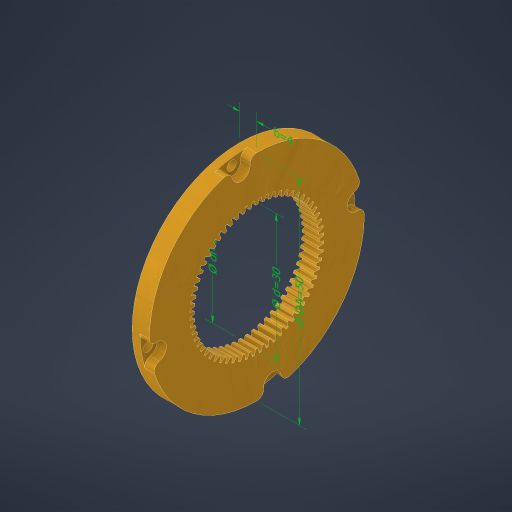
# Autodesk Inventor part: 60z
Saved by Autodesk Inventor 2024.1 (Build 281209000, 209)
## iProperties
Category: PARTsolutions
Company: MAEDLER
Created: 2023-10-17
Part Number: 60z
Material: Generic
Catalog Web Link: www.cadenas.de
Description: MAE-IZK-M0.5-MS58-Straight-Toothed Internal Gears Made from Brass MS58, Module 0,5
Vendor: MAEDLER
Document SubType Name: Modeling
Designer: psAdmin
Manufacturer: MAEDLER
Mass: 42 g
Surface Area: 39.2862 cm^2
Volume: 5.00767 cm^3
Density: 1 g/cm^3
Appearance: Schweißnaht - Messing
PSOL_IDENT_0: {$CADENAS_DATA/23d-libs/maedler/antriebselemente/innenzahnkraenze/innenzahnkr_m0_5_ms58.prj},167 {VT
PSOL_IDENT_1: YP=3D},{NB=26146000},{LINA=26146000},{NN=MAE-IZK-M0.5-MS58},{DATE=12.10.2023 13:22:54},{GEOMDATE=09.
PSOL_IDENT_2: 07.2023 12:07:43},{VERSION=},{LINEID=50},{WBVAR=},{WBNUMERIC=}  {NB=26146000},{LINA=26146000},{KT=DU
PSOL_IDENT_3: MMY},{ARTNR=26146000},{WEBSHOP=Produktdetails / Katalogseite / Montageanleitung},{MAT=Messing MS58 (
PSOL_IDENT_4: 2.0401)},{M=0.5},{Z=60},{B=4},{D=30.0},{DI=29.0},{DA=50},{GEW=42},{ZTN=84839089},{DIST=1.800}
NB: 26146000
NN: MAE-IZK-M0.5-MS58
NT: Straight-Toothed Internal Gears Made from Brass MS58, Module 0,5
NBSYN: $ARTNR.
LINA: 26146000
CATALOG: Mädler
ARTNR: 26146000
WEBSHOP: Product details / Catalogue page / Assembly instructions
MAT: Brass Ms58 (2.0401)
M: 0.5
Z: 60
B: 4
D: 30
DI: 29
DA: 50
GEW: 42
ZTN: 84839089
SUPPLIER: MAEDLER
ARTICLENO: 26146000
BOMINFO: 26146000
CREATOR: CADENAS GmbH
Title: 26146000
Author: Cadenas PARTsolutions
Comments: Straight-Toothed Internal Gears Made from Brass MS58, Module 0,5
Autodesk Inventor part; units mm, degrees
ref_plane "YZ Plane" through (0, 0, 0) normal (1, 0, 0) x (0, 1, 0)
ref_plane "XZ Plane" through (0, 0, 0) normal (0, 1, 0) x (-1, 0, 0)
ref_plane "XY Plane" through (0, 0, 0) normal (0, 0, 1) x (1, 0, 0)
sketch "Skizze_1" plane through (0, 0, 0) normal (1, 0, 0) x (0, 1, 0)
  circle A0 centre (0, 0) radius 25
  line L0 (0.5705, 15.6146) -> (0.25, 14.4978)
  arc A1 (0.25, 14.4978) -> (-0.25, 14.4978) centre (0, 0) ccw
  line L1 (-0.25, 14.4978) -> (-0.5705, 15.6146)
  arc A2 (-0.5705, 15.6146) -> (-1.0648, 15.5887) centre (0, 0) ccw
  line L2 (-1.0648, 15.5887) -> (-1.2668, 14.4446)
  arc A3 (-1.2668, 14.4446) -> (-1.7641, 14.3923) centre (0, 0) ccw
  line L3 (-1.7641, 14.3923) -> (-2.1996, 15.4694)
  arc A4 (-2.1996, 15.4694) -> (-2.6884, 15.392) centre (0, 0) ccw
  line L4 (-2.6884, 15.392) -> (-2.7697, 14.233)
  arc A5 (-2.7697, 14.233) -> (-3.2588, 14.1291) centre (0, 0) ccw
  line L5 (-3.2588, 14.1291) -> (-3.8045, 15.1547)
  arc A6 (-3.8045, 15.1547) -> (-4.2826, 15.0267) centre (0, 0) ccw
  line L6 (-4.2826, 15.0267) -> (-4.2423, 13.8655)
  arc A7 (-4.2423, 13.8655) -> (-4.7178, 13.711) centre (0, 0) ccw
  line L7 (-4.7178, 13.711) -> (-5.3678, 14.674)
  arc A8 (-5.3678, 14.674) -> (-5.8298, 14.4967) centre (0, 0) ccw
  line L8 (-5.8298, 14.4967) -> (-5.6684, 13.3461)
  arc A9 (-5.6684, 13.3461) -> (-6.1252, 13.1428) centre (0, 0) ccw
  line L9 (-6.1252, 13.1428) -> (-6.8722, 14.0326)
  arc A10 (-6.8722, 14.0326) -> (-7.3132, 13.8079) centre (0, 0) ccw
  line L10 (-7.3132, 13.8079) -> (-7.0324, 12.6805)
  arc A11 (-7.0324, 12.6805) -> (-7.4654, 12.4305) centre (0, 0) ccw
  line L11 (-7.4654, 12.4305) -> (-8.3014, 13.2374)
  arc A12 (-8.3014, 13.2374) -> (-8.7165, 12.9678) centre (0, 0) ccw
  line L12 (-8.7165, 12.9678) -> (-8.3194, 11.8759)
  arc A13 (-8.3194, 11.8759) -> (-8.7239, 11.5821) centre (0, 0) ccw
  line L13 (-8.7239, 11.5821) -> (-9.6396, 12.2971)
  arc A14 (-9.6396, 12.2971) -> (-10.0242, 11.9857) centre (0, 0) ccw
  line L14 (-10.0242, 11.9857) -> (-9.5152, 10.9413)
  arc A15 (-9.5152, 10.9413) -> (-9.8867, 10.6067) centre (0, 0) ccw
  line L15 (-9.8867, 10.6067) -> (-10.8722, 11.2221)
  arc A16 (-10.8722, 11.2221) -> (-11.2221, 10.8722) centre (0, 0) ccw
  line L16 (-11.2221, 10.8722) -> (-10.6067, 9.8867)
  arc A17 (-10.6067, 9.8867) -> (-10.9413, 9.5152) centre (0, 0) ccw
  line L17 (-10.9413, 9.5152) -> (-11.9857, 10.0242)
  arc A18 (-11.9857, 10.0242) -> (-12.2971, 9.6396) centre (0, 0) ccw
  line L18 (-12.2971, 9.6396) -> (-11.5821, 8.7239)
  arc A19 (-11.5821, 8.7239) -> (-11.8759, 8.3194) centre (0, 0) ccw
  line L19 (-11.8759, 8.3194) -> (-12.9678, 8.7165)
  arc A20 (-12.9678, 8.7165) -> (-13.2374, 8.3014) centre (0, 0) ccw
  line L20 (-13.2374, 8.3014) -> (-12.4305, 7.4654)
  arc A21 (-12.4305, 7.4654) -> (-12.6805, 7.0324) centre (0, 0) ccw
  line L21 (-12.6805, 7.0324) -> (-13.8079, 7.3132)
  arc A22 (-13.8079, 7.3132) -> (-14.0326, 6.8722) centre (0, 0) ccw
  line L22 (-14.0326, 6.8722) -> (-13.1428, 6.1252)
  arc A23 (-13.1428, 6.1252) -> (-13.3461, 5.6684) centre (0, 0) ccw
  line L23 (-13.3461, 5.6684) -> (-14.4967, 5.8298)
  arc A24 (-14.4967, 5.8298) -> (-14.674, 5.3678) centre (0, 0) ccw
  line L24 (-14.674, 5.3678) -> (-13.711, 4.7178)
  arc A25 (-13.711, 4.7178) -> (-13.8655, 4.2423) centre (0, 0) ccw
  line L25 (-13.8655, 4.2423) -> (-15.0267, 4.2826)
  arc A26 (-15.0267, 4.2826) -> (-15.1547, 3.8045) centre (0, 0) ccw
  line L26 (-15.1547, 3.8045) -> (-14.1291, 3.2588)
  arc A27 (-14.1291, 3.2588) -> (-14.233, 2.7697) centre (0, 0) ccw
  line L27 (-14.233, 2.7697) -> (-15.392, 2.6884)
  arc A28 (-15.392, 2.6884) -> (-15.4694, 2.1996) centre (0, 0) ccw
  line L28 (-15.4694, 2.1996) -> (-14.3923, 1.7641)
  arc A29 (-14.3923, 1.7641) -> (-14.4446, 1.2668) centre (0, 0) ccw
  line L29 (-14.4446, 1.2668) -> (-15.5887, 1.0648)
  arc A30 (-15.5887, 1.0648) -> (-15.6146, 0.5705) centre (0, 0) ccw
  line L30 (-15.6146, 0.5705) -> (-14.4978, 0.25)
  arc A31 (-14.4978, 0.25) -> (-14.4978, -0.25) centre (0, 0) ccw
  line L31 (-14.4978, -0.25) -> (-15.6146, -0.5705)
  arc A32 (-15.6146, -0.5705) -> (-15.5887, -1.0648) centre (0, 0) ccw
  line L32 (-15.5887, -1.0648) -> (-14.4446, -1.2668)
  arc A33 (-14.4446, -1.2668) -> (-14.3923, -1.7641) centre (0, 0) ccw
  line L33 (-14.3923, -1.7641) -> (-15.4694, -2.1996)
  arc A34 (-15.4694, -2.1996) -> (-15.392, -2.6884) centre (0, 0) ccw
  line L34 (-15.392, -2.6884) -> (-14.233, -2.7697)
  arc A35 (-14.233, -2.7697) -> (-14.1291, -3.2588) centre (0, 0) ccw
  line L35 (-14.1291, -3.2588) -> (-15.1547, -3.8045)
  arc A36 (-15.1547, -3.8045) -> (-15.0267, -4.2826) centre (0, 0) ccw
  line L36 (-15.0267, -4.2826) -> (-13.8655, -4.2423)
  arc A37 (-13.8655, -4.2423) -> (-13.711, -4.7178) centre (0, 0) ccw
  line L37 (-13.711, -4.7178) -> (-14.674, -5.3678)
  arc A38 (-14.674, -5.3678) -> (-14.4967, -5.8298) centre (0, 0) ccw
  line L38 (-14.4967, -5.8298) -> (-13.3461, -5.6684)
  arc A39 (-13.3461, -5.6684) -> (-13.1428, -6.1252) centre (0, 0) ccw
  line L39 (-13.1428, -6.1252) -> (-14.0326, -6.8722)
  arc A40 (-14.0326, -6.8722) -> (-13.8079, -7.3132) centre (0, 0) ccw
  line L40 (-13.8079, -7.3132) -> (-12.6805, -7.0324)
  arc A41 (-12.6805, -7.0324) -> (-12.4305, -7.4654) centre (0, 0) ccw
  line L41 (-12.4305, -7.4654) -> (-13.2374, -8.3014)
  arc A42 (-13.2374, -8.3014) -> (-12.9678, -8.7165) centre (0, 0) ccw
  line L42 (-12.9678, -8.7165) -> (-11.8759, -8.3194)
  arc A43 (-11.8759, -8.3194) -> (-11.5821, -8.7239) centre (0, 0) ccw
  line L43 (-11.5821, -8.7239) -> (-12.2971, -9.6396)
  arc A44 (-12.2971, -9.6396) -> (-11.9857, -10.0242) centre (0, 0) ccw
  line L44 (-11.9857, -10.0242) -> (-10.9413, -9.5152)
  arc A45 (-10.9413, -9.5152) -> (-10.6067, -9.8867) centre (0, 0) ccw
  line L45 (-10.6067, -9.8867) -> (-11.2221, -10.8722)
  arc A46 (-11.2221, -10.8722) -> (-10.8722, -11.2221) centre (0, 0) ccw
  line L46 (-10.8722, -11.2221) -> (-9.8867, -10.6067)
  arc A47 (-9.8867, -10.6067) -> (-9.5152, -10.9413) centre (0, 0) ccw
  line L47 (-9.5152, -10.9413) -> (-10.0242, -11.9857)
  arc A48 (-10.0242, -11.9857) -> (-9.6396, -12.2971) centre (0, 0) ccw
  line L48 (-9.6396, -12.2971) -> (-8.7239, -11.5821)
  arc A49 (-8.7239, -11.5821) -> (-8.3194, -11.8759) centre (0, 0) ccw
  line L49 (-8.3194, -11.8759) -> (-8.7165, -12.9678)
  arc A50 (-8.7165, -12.9678) -> (-8.3014, -13.2374) centre (0, 0) ccw
  line L50 (-8.3014, -13.2374) -> (-7.4654, -12.4305)
  arc A51 (-7.4654, -12.4305) -> (-7.0324, -12.6805) centre (0, 0) ccw
  line L51 (-7.0324, -12.6805) -> (-7.3132, -13.8079)
  arc A52 (-7.3132, -13.8079) -> (-6.8722, -14.0326) centre (0, 0) ccw
  line L52 (-6.8722, -14.0326) -> (-6.1252, -13.1428)
  arc A53 (-6.1252, -13.1428) -> (-5.6684, -13.3461) centre (0, 0) ccw
  line L53 (-5.6684, -13.3461) -> (-5.8298, -14.4967)
  arc A54 (-5.8298, -14.4967) -> (-5.3678, -14.674) centre (0, 0) ccw
  line L54 (-5.3678, -14.674) -> (-4.7178, -13.711)
  arc A55 (-4.7178, -13.711) -> (-4.2423, -13.8655) centre (0, 0) ccw
  line L55 (-4.2423, -13.8655) -> (-4.2826, -15.0267)
  arc A56 (-4.2826, -15.0267) -> (-3.8045, -15.1547) centre (0, 0) ccw
  line L56 (-3.8045, -15.1547) -> (-3.2588, -14.1291)
  arc A57 (-3.2588, -14.1291) -> (-2.7697, -14.233) centre (0, 0) ccw
  line L57 (-2.7697, -14.233) -> (-2.6884, -15.392)
  arc A58 (-2.6884, -15.392) -> (-2.1996, -15.4694) centre (0, 0) ccw
  line L58 (-2.1996, -15.4694) -> (-1.7641, -14.3923)
  arc A59 (-1.7641, -14.3923) -> (-1.2668, -14.4446) centre (0, 0) ccw
  line L59 (-1.2668, -14.4446) -> (-1.0648, -15.5887)
  arc A60 (-1.0648, -15.5887) -> (-0.5705, -15.6146) centre (0, 0) ccw
  line L60 (-0.5705, -15.6146) -> (-0.25, -14.4978)
  arc A61 (-0.25, -14.4978) -> (0.25, -14.4978) centre (0, 0) ccw
  line L61 (0.25, -14.4978) -> (0.5705, -15.6146)
  arc A62 (0.5705, -15.6146) -> (1.0648, -15.5887) centre (0, 0) ccw
  line L62 (1.0648, -15.5887) -> (1.2668, -14.4446)
  arc A63 (1.2668, -14.4446) -> (1.7641, -14.3923) centre (0, 0) ccw
  line L63 (1.7641, -14.3923) -> (2.1996, -15.4694)
  arc A64 (2.1996, -15.4694) -> (2.6884, -15.392) centre (0, 0) ccw
  line L64 (2.6884, -15.392) -> (2.7697, -14.233)
  arc A65 (2.7697, -14.233) -> (3.2588, -14.1291) centre (0, 0) ccw
  line L65 (3.2588, -14.1291) -> (3.8045, -15.1547)
  arc A66 (3.8045, -15.1547) -> (4.2826, -15.0267) centre (0, 0) ccw
  line L66 (4.2826, -15.0267) -> (4.2423, -13.8655)
  arc A67 (4.2423, -13.8655) -> (4.7178, -13.711) centre (0, 0) ccw
  line L67 (4.7178, -13.711) -> (5.3678, -14.674)
  arc A68 (5.3678, -14.674) -> (5.8298, -14.4967) centre (0, 0) ccw
  line L68 (5.8298, -14.4967) -> (5.6684, -13.3461)
  arc A69 (5.6684, -13.3461) -> (6.1252, -13.1428) centre (0, 0) ccw
  line L69 (6.1252, -13.1428) -> (6.8722, -14.0326)
  arc A70 (6.8722, -14.0326) -> (7.3132, -13.8079) centre (0, 0) ccw
  line L70 (7.3132, -13.8079) -> (7.0324, -12.6805)
  arc A71 (7.0324, -12.6805) -> (7.4654, -12.4305) centre (0, 0) ccw
  line L71 (7.4654, -12.4305) -> (8.3014, -13.2374)
  arc A72 (8.3014, -13.2374) -> (8.7165, -12.9678) centre (0, 0) ccw
  line L72 (8.7165, -12.9678) -> (8.3194, -11.8759)
  arc A73 (8.3194, -11.8759) -> (8.7239, -11.5821) centre (0, 0) ccw
  line L73 (8.7239, -11.5821) -> (9.6396, -12.2971)
  arc A74 (9.6396, -12.2971) -> (10.0242, -11.9857) centre (0, 0) ccw
  line L74 (10.0242, -11.9857) -> (9.5152, -10.9413)
  arc A75 (9.5152, -10.9413) -> (9.8867, -10.6067) centre (0, 0) ccw
  line L75 (9.8867, -10.6067) -> (10.8722, -11.2221)
  arc A76 (10.8722, -11.2221) -> (11.2221, -10.8722) centre (0, 0) ccw
  line L76 (11.2221, -10.8722) -> (10.6067, -9.8867)
  arc A77 (10.6067, -9.8867) -> (10.9413, -9.5152) centre (0, 0) ccw
  line L77 (10.9413, -9.5152) -> (11.9857, -10.0242)
  arc A78 (11.9857, -10.0242) -> (12.2971, -9.6396) centre (0, 0) ccw
  line L78 (12.2971, -9.6396) -> (11.5821, -8.7239)
  arc A79 (11.5821, -8.7239) -> (11.8759, -8.3194) centre (0, 0) ccw
  line L79 (11.8759, -8.3194) -> (12.9678, -8.7165)
  arc A80 (12.9678, -8.7165) -> (13.2374, -8.3014) centre (0, 0) ccw
  line L80 (13.2374, -8.3014) -> (12.4305, -7.4654)
  arc A81 (12.4305, -7.4654) -> (12.6805, -7.0324) centre (0, 0) ccw
  line L81 (12.6805, -7.0324) -> (13.8079, -7.3132)
  arc A82 (13.8079, -7.3132) -> (14.0326, -6.8722) centre (0, 0) ccw
  line L82 (14.0326, -6.8722) -> (13.1428, -6.1252)
  arc A83 (13.1428, -6.1252) -> (13.3461, -5.6684) centre (0, 0) ccw
  line L83 (13.3461, -5.6684) -> (14.4967, -5.8298)
  arc A84 (14.4967, -5.8298) -> (14.674, -5.3678) centre (0, 0) ccw
  line L84 (14.674, -5.3678) -> (13.711, -4.7178)
  arc A85 (13.711, -4.7178) -> (13.8655, -4.2423) centre (0, 0) ccw
  line L85 (13.8655, -4.2423) -> (15.0267, -4.2826)
  arc A86 (15.0267, -4.2826) -> (15.1547, -3.8045) centre (0, 0) ccw
  line L86 (15.1547, -3.8045) -> (14.1291, -3.2588)
  arc A87 (14.1291, -3.2588) -> (14.233, -2.7697) centre (0, 0) ccw
  line L87 (14.233, -2.7697) -> (15.392, -2.6884)
  arc A88 (15.392, -2.6884) -> (15.4694, -2.1996) centre (0, 0) ccw
  line L88 (15.4694, -2.1996) -> (14.3923, -1.7641)
  arc A89 (14.3923, -1.7641) -> (14.4446, -1.2668) centre (0, 0) ccw
  line L89 (14.4446, -1.2668) -> (15.5887, -1.0648)
  arc A90 (15.5887, -1.0648) -> (15.6146, -0.5705) centre (0, 0) ccw
  line L90 (15.6146, -0.5705) -> (14.4978, -0.25)
  arc A91 (14.4978, -0.25) -> (14.4978, 0.25) centre (0, 0) ccw
  line L91 (14.4978, 0.25) -> (15.6146, 0.5705)
  arc A92 (15.6146, 0.5705) -> (15.5887, 1.0648) centre (0, 0) ccw
  line L92 (15.5887, 1.0648) -> (14.4446, 1.2668)
  arc A93 (14.4446, 1.2668) -> (14.3923, 1.7641) centre (0, 0) ccw
  line L93 (14.3923, 1.7641) -> (15.4694, 2.1996)
  arc A94 (15.4694, 2.1996) -> (15.392, 2.6884) centre (0, 0) ccw
  line L94 (15.392, 2.6884) -> (14.233, 2.7697)
  arc A95 (14.233, 2.7697) -> (14.1291, 3.2588) centre (0, 0) ccw
  line L95 (14.1291, 3.2588) -> (15.1547, 3.8045)
  arc A96 (15.1547, 3.8045) -> (15.0267, 4.2826) centre (0, 0) ccw
  line L96 (15.0267, 4.2826) -> (13.8655, 4.2423)
  arc A97 (13.8655, 4.2423) -> (13.711, 4.7178) centre (0, 0) ccw
  line L97 (13.711, 4.7178) -> (14.674, 5.3678)
  arc A98 (14.674, 5.3678) -> (14.4967, 5.8298) centre (0, 0) ccw
  line L98 (14.4967, 5.8298) -> (13.3461, 5.6684)
  arc A99 (13.3461, 5.6684) -> (13.1428, 6.1252) centre (0, 0) ccw
  line L99 (13.1428, 6.1252) -> (14.0326, 6.8722)
  arc A100 (14.0326, 6.8722) -> (13.8079, 7.3132) centre (0, 0) ccw
  line L100 (13.8079, 7.3132) -> (12.6805, 7.0324)
  arc A101 (12.6805, 7.0324) -> (12.4305, 7.4654) centre (0, 0) ccw
  line L101 (12.4305, 7.4654) -> (13.2374, 8.3014)
  arc A102 (13.2374, 8.3014) -> (12.9678, 8.7165) centre (0, 0) ccw
  line L102 (12.9678, 8.7165) -> (11.8759, 8.3194)
  arc A103 (11.8759, 8.3194) -> (11.5821, 8.7239) centre (0, 0) ccw
  line L103 (11.5821, 8.7239) -> (12.2971, 9.6396)
  arc A104 (12.2971, 9.6396) -> (11.9857, 10.0242) centre (0, 0) ccw
  line L104 (11.9857, 10.0242) -> (10.9413, 9.5152)
  arc A105 (10.9413, 9.5152) -> (10.6067, 9.8867) centre (0, 0) ccw
  line L105 (10.6067, 9.8867) -> (11.2221, 10.8722)
  arc A106 (11.2221, 10.8722) -> (10.8722, 11.2221) centre (0, 0) ccw
  line L106 (10.8722, 11.2221) -> (9.8867, 10.6067)
  arc A107 (9.8867, 10.6067) -> (9.5152, 10.9413) centre (0, 0) ccw
  line L107 (9.5152, 10.9413) -> (10.0242, 11.9857)
  arc A108 (10.0242, 11.9857) -> (9.6396, 12.2971) centre (0, 0) ccw
  line L108 (9.6396, 12.2971) -> (8.7239, 11.5821)
  arc A109 (8.7239, 11.5821) -> (8.3194, 11.8759) centre (0, 0) ccw
  line L109 (8.3194, 11.8759) -> (8.7165, 12.9678)
  arc A110 (8.7165, 12.9678) -> (8.3014, 13.2374) centre (0, 0) ccw
  line L110 (8.3014, 13.2374) -> (7.4654, 12.4305)
  arc A111 (7.4654, 12.4305) -> (7.0324, 12.6805) centre (0, 0) ccw
  line L111 (7.0324, 12.6805) -> (7.3132, 13.8079)
  arc A112 (7.3132, 13.8079) -> (6.8722, 14.0326) centre (0, 0) ccw
  line L112 (6.8722, 14.0326) -> (6.1252, 13.1428)
  arc A113 (6.1252, 13.1428) -> (5.6684, 13.3461) centre (0, 0) ccw
  line L113 (5.6684, 13.3461) -> (5.8298, 14.4967)
  arc A114 (5.8298, 14.4967) -> (5.3678, 14.674) centre (0, 0) ccw
  line L114 (5.3678, 14.674) -> (4.7178, 13.711)
  arc A115 (4.7178, 13.711) -> (4.2423, 13.8655) centre (0, 0) ccw
  line L115 (4.2423, 13.8655) -> (4.2826, 15.0267)
  arc A116 (4.2826, 15.0267) -> (3.8045, 15.1547) centre (0, 0) ccw
  line L116 (3.8045, 15.1547) -> (3.2588, 14.1291)
  arc A117 (3.2588, 14.1291) -> (2.7697, 14.233) centre (0, 0) ccw
  line L117 (2.7697, 14.233) -> (2.6884, 15.392)
  arc A118 (2.6884, 15.392) -> (2.1996, 15.4694) centre (0, 0) ccw
  line L118 (2.1996, 15.4694) -> (1.7641, 14.3923)
  arc A119 (1.7641, 14.3923) -> (1.2668, 14.4446) centre (0, 0) ccw
  line L119 (1.2668, 14.4446) -> (1.0648, 15.5887)
  arc A120 (1.0648, 15.5887) -> (0.5705, 15.6146) centre (0, 0) ccw
  constraints: 240 end point, 240 point on circle, 121 centre point
extrude "Extrusion1" add sketch "Skizze_1" along normal mid plane 4
sketch "Skizze4" plane through (2, 0, 0) normal (1, 0, 0) x (0, 0, -1)
  line L0 (0.5705, 15.6146) -> (0.25, 14.4978)
  arc A0 (0.25, 14.4978) -> (-0.25, 14.4978) centre (0, 0) ccw
  line L1 (-0.25, 14.4978) -> (-0.5705, 15.6146)
  arc A1 (-0.5705, 15.6146) -> (-1.0648, 15.5887) centre (0, 0) ccw
  line L2 (-1.0648, 15.5887) -> (-1.2668, 14.4446)
  arc A2 (-1.2668, 14.4446) -> (-1.7641, 14.3923) centre (0, 0) ccw
  line L3 (-1.7641, 14.3923) -> (-2.1996, 15.4694)
  arc A3 (-2.1996, 15.4694) -> (-2.6884, 15.392) centre (0, 0) ccw
  line L4 (-2.6884, 15.392) -> (-2.7697, 14.233)
  arc A4 (-2.7697, 14.233) -> (-3.2588, 14.1291) centre (0, 0) ccw
  line L5 (-3.2588, 14.1291) -> (-3.8045, 15.1547)
  arc A5 (-3.8045, 15.1547) -> (-4.2826, 15.0267) centre (0, 0) ccw
  line L6 (-4.2826, 15.0267) -> (-4.2423, 13.8655)
  arc A6 (-4.2423, 13.8655) -> (-4.7178, 13.711) centre (0, 0) ccw
  line L7 (-4.7178, 13.711) -> (-5.3678, 14.674)
  arc A7 (-5.3678, 14.674) -> (-5.8298, 14.4967) centre (0, 0) ccw
  line L8 (-5.8298, 14.4967) -> (-5.6684, 13.3461)
  arc A8 (-5.6684, 13.3461) -> (-6.1252, 13.1428) centre (0, 0) ccw
  line L9 (-6.1252, 13.1428) -> (-6.8722, 14.0326)
  arc A9 (-6.8722, 14.0326) -> (-7.3132, 13.8079) centre (0, 0) ccw
  line L10 (-7.3132, 13.8079) -> (-7.0324, 12.6805)
  arc A10 (-7.0324, 12.6805) -> (-7.4654, 12.4305) centre (0, 0) ccw
  line L11 (-7.4654, 12.4305) -> (-8.3014, 13.2374)
  arc A11 (-8.3014, 13.2374) -> (-8.7165, 12.9678) centre (0, 0) ccw
  line L12 (-8.7165, 12.9678) -> (-8.3194, 11.8759)
  arc A12 (-8.3194, 11.8759) -> (-8.7239, 11.5821) centre (0, 0) ccw
  line L13 (-8.7239, 11.5821) -> (-9.6396, 12.2971)
  arc A13 (-9.6396, 12.2971) -> (-10.0242, 11.9857) centre (0, 0) ccw
  line L14 (-10.0242, 11.9857) -> (-9.5152, 10.9413)
  arc A14 (-9.5152, 10.9413) -> (-9.8867, 10.6067) centre (0, 0) ccw
  line L15 (-9.8867, 10.6067) -> (-10.8722, 11.2221)
  arc A15 (-10.8722, 11.2221) -> (-11.2221, 10.8722) centre (0, 0) ccw
  line L16 (-11.2221, 10.8722) -> (-10.6067, 9.8867)
  arc A16 (-10.6067, 9.8867) -> (-10.9413, 9.5152) centre (0, 0) ccw
  line L17 (-10.9413, 9.5152) -> (-11.9857, 10.0242)
  arc A17 (-11.9857, 10.0242) -> (-12.2971, 9.6396) centre (0, 0) ccw
  line L18 (-12.2971, 9.6396) -> (-11.5821, 8.7239)
  arc A18 (-11.5821, 8.7239) -> (-11.8759, 8.3194) centre (0, 0) ccw
  line L19 (-11.8759, 8.3194) -> (-12.9678, 8.7165)
  arc A19 (-12.9678, 8.7165) -> (-13.2374, 8.3014) centre (0, 0) ccw
  line L20 (-13.2374, 8.3014) -> (-12.4305, 7.4654)
  arc A20 (-12.4305, 7.4654) -> (-12.6805, 7.0324) centre (0, 0) ccw
  line L21 (-12.6805, 7.0324) -> (-13.8079, 7.3132)
  arc A21 (-13.8079, 7.3132) -> (-14.0326, 6.8722) centre (0, 0) ccw
  line L22 (-14.0326, 6.8722) -> (-13.1428, 6.1252)
  arc A22 (-13.1428, 6.1252) -> (-13.3461, 5.6684) centre (0, 0) ccw
  line L23 (-13.3461, 5.6684) -> (-14.4967, 5.8298)
  arc A23 (-14.4967, 5.8298) -> (-14.674, 5.3678) centre (0, 0) ccw
  line L24 (-14.674, 5.3678) -> (-13.711, 4.7178)
  arc A24 (-13.711, 4.7178) -> (-13.8655, 4.2423) centre (0, 0) ccw
  line L25 (-13.8655, 4.2423) -> (-15.0267, 4.2826)
  arc A25 (-15.0267, 4.2826) -> (-15.1547, 3.8045) centre (0, 0) ccw
  line L26 (-15.1547, 3.8045) -> (-14.1291, 3.2588)
  arc A26 (-14.1291, 3.2588) -> (-14.233, 2.7697) centre (0, 0) ccw
  line L27 (-14.233, 2.7697) -> (-15.392, 2.6884)
  arc A27 (-15.392, 2.6884) -> (-15.4694, 2.1996) centre (0, 0) ccw
  line L28 (-15.4694, 2.1996) -> (-14.3923, 1.7641)
  arc A28 (-14.3923, 1.7641) -> (-14.4446, 1.2668) centre (0, 0) ccw
  line L29 (-14.4446, 1.2668) -> (-15.5887, 1.0648)
  arc A29 (-15.5887, 1.0648) -> (-15.6146, 0.5705) centre (0, 0) ccw
  line L30 (-15.6146, 0.5705) -> (-14.4978, 0.25)
  arc A30 (-14.4978, 0.25) -> (-14.4978, -0.25) centre (0, 0) ccw
  line L31 (-14.4978, -0.25) -> (-15.6146, -0.5705)
  arc A31 (-15.6146, -0.5705) -> (-15.5887, -1.0648) centre (0, 0) ccw
  line L32 (-15.5887, -1.0648) -> (-14.4446, -1.2668)
  arc A32 (-14.4446, -1.2668) -> (-14.3923, -1.7641) centre (0, 0) ccw
  line L33 (-14.3923, -1.7641) -> (-15.4694, -2.1996)
  arc A33 (-15.4694, -2.1996) -> (-15.392, -2.6884) centre (0, 0) ccw
  line L34 (-15.392, -2.6884) -> (-14.233, -2.7697)
  arc A34 (-14.233, -2.7697) -> (-14.1291, -3.2588) centre (0, 0) ccw
  line L35 (-14.1291, -3.2588) -> (-15.1547, -3.8045)
  arc A35 (-15.1547, -3.8045) -> (-15.0267, -4.2826) centre (0, 0) ccw
  line L36 (-15.0267, -4.2826) -> (-13.8655, -4.2423)
  arc A36 (-13.8655, -4.2423) -> (-13.711, -4.7178) centre (0, 0) ccw
  line L37 (-13.711, -4.7178) -> (-14.674, -5.3678)
  arc A37 (-14.674, -5.3678) -> (-14.4967, -5.8298) centre (0, 0) ccw
  line L38 (-14.4967, -5.8298) -> (-13.3461, -5.6684)
  arc A38 (-13.3461, -5.6684) -> (-13.1428, -6.1252) centre (0, 0) ccw
  line L39 (-13.1428, -6.1252) -> (-14.0326, -6.8722)
  arc A39 (-14.0326, -6.8722) -> (-13.8079, -7.3132) centre (0, 0) ccw
  line L40 (-13.8079, -7.3132) -> (-12.6805, -7.0324)
  arc A40 (-12.6805, -7.0324) -> (-12.4305, -7.4654) centre (0, 0) ccw
  line L41 (-12.4305, -7.4654) -> (-13.2374, -8.3014)
  arc A41 (-13.2374, -8.3014) -> (-12.9678, -8.7165) centre (0, 0) ccw
  line L42 (-12.9678, -8.7165) -> (-11.8759, -8.3194)
  arc A42 (-11.8759, -8.3194) -> (-11.5821, -8.7239) centre (0, 0) ccw
  line L43 (-11.5821, -8.7239) -> (-12.2971, -9.6396)
  arc A43 (-12.2971, -9.6396) -> (-11.9857, -10.0242) centre (0, 0) ccw
  line L44 (-11.9857, -10.0242) -> (-10.9413, -9.5152)
  arc A44 (-10.9413, -9.5152) -> (-10.6067, -9.8867) centre (0, 0) ccw
  line L45 (-10.6067, -9.8867) -> (-11.2221, -10.8722)
  arc A45 (-11.2221, -10.8722) -> (-10.8722, -11.2221) centre (0, 0) ccw
  line L46 (-10.8722, -11.2221) -> (-9.8867, -10.6067)
  arc A46 (-9.8867, -10.6067) -> (-9.5152, -10.9413) centre (0, 0) ccw
  line L47 (-9.5152, -10.9413) -> (-10.0242, -11.9857)
  arc A47 (-10.0242, -11.9857) -> (-9.6396, -12.2971) centre (0, 0) ccw
  line L48 (-9.6396, -12.2971) -> (-8.7239, -11.5821)
  arc A48 (-8.7239, -11.5821) -> (-8.3194, -11.8759) centre (0, 0) ccw
  line L49 (-8.3194, -11.8759) -> (-8.7165, -12.9678)
  arc A49 (-8.7165, -12.9678) -> (-8.3014, -13.2374) centre (0, 0) ccw
  line L50 (-8.3014, -13.2374) -> (-7.4654, -12.4305)
  arc A50 (-7.4654, -12.4305) -> (-7.0324, -12.6805) centre (0, 0) ccw
  line L51 (-7.0324, -12.6805) -> (-7.3132, -13.8079)
  arc A51 (-7.3132, -13.8079) -> (-6.8722, -14.0326) centre (0, 0) ccw
  line L52 (-6.8722, -14.0326) -> (-6.1252, -13.1428)
  arc A52 (-6.1252, -13.1428) -> (-5.6684, -13.3461) centre (0, 0) ccw
  line L53 (-5.6684, -13.3461) -> (-5.8298, -14.4967)
  arc A53 (-5.8298, -14.4967) -> (-5.3678, -14.674) centre (0, 0) ccw
  line L54 (-5.3678, -14.674) -> (-4.7178, -13.711)
  arc A54 (-4.7178, -13.711) -> (-4.2423, -13.8655) centre (0, 0) ccw
  line L55 (-4.2423, -13.8655) -> (-4.2826, -15.0267)
  arc A55 (-4.2826, -15.0267) -> (-3.8045, -15.1547) centre (0, 0) ccw
  line L56 (-3.8045, -15.1547) -> (-3.2588, -14.1291)
  arc A56 (-3.2588, -14.1291) -> (-2.7697, -14.233) centre (0, 0) ccw
  line L57 (-2.7697, -14.233) -> (-2.6884, -15.392)
  arc A57 (-2.6884, -15.392) -> (-2.1996, -15.4694) centre (0, 0) ccw
  line L58 (-2.1996, -15.4694) -> (-1.7641, -14.3923)
  arc A58 (-1.7641, -14.3923) -> (-1.2668, -14.4446) centre (0, 0) ccw
  line L59 (-1.2668, -14.4446) -> (-1.0648, -15.5887)
  arc A59 (-1.0648, -15.5887) -> (-0.5705, -15.6146) centre (0, 0) ccw
  line L60 (-0.5705, -15.6146) -> (-0.25, -14.4978)
  arc A60 (-0.25, -14.4978) -> (0.25, -14.4978) centre (0, 0) ccw
  line L61 (0.25, -14.4978) -> (0.5705, -15.6146)
  arc A61 (0.5705, -15.6146) -> (1.0648, -15.5887) centre (0, 0) ccw
  line L62 (1.0648, -15.5887) -> (1.2668, -14.4446)
  arc A62 (1.2668, -14.4446) -> (1.7641, -14.3923) centre (0, 0) ccw
  line L63 (1.7641, -14.3923) -> (2.1996, -15.4694)
  arc A63 (2.1996, -15.4694) -> (2.6884, -15.392) centre (0, 0) ccw
  line L64 (2.6884, -15.392) -> (2.7697, -14.233)
  arc A64 (2.7697, -14.233) -> (3.2588, -14.1291) centre (0, 0) ccw
  line L65 (3.2588, -14.1291) -> (3.8045, -15.1547)
  arc A65 (3.8045, -15.1547) -> (4.2826, -15.0267) centre (0, 0) ccw
  line L66 (4.2826, -15.0267) -> (4.2423, -13.8655)
  arc A66 (4.2423, -13.8655) -> (4.7178, -13.711) centre (0, 0) ccw
  line L67 (4.7178, -13.711) -> (5.3678, -14.674)
  arc A67 (5.3678, -14.674) -> (5.8298, -14.4967) centre (0, 0) ccw
  line L68 (5.8298, -14.4967) -> (5.6684, -13.3461)
  arc A68 (5.6684, -13.3461) -> (6.1252, -13.1428) centre (0, 0) ccw
  line L69 (6.1252, -13.1428) -> (6.8722, -14.0326)
  arc A69 (6.8722, -14.0326) -> (7.3132, -13.8079) centre (0, 0) ccw
  line L70 (7.3132, -13.8079) -> (7.0324, -12.6805)
  arc A70 (7.0324, -12.6805) -> (7.4654, -12.4305) centre (0, 0) ccw
  line L71 (7.4654, -12.4305) -> (8.3014, -13.2374)
  arc A71 (8.3014, -13.2374) -> (8.7165, -12.9678) centre (0, 0) ccw
  line L72 (8.7165, -12.9678) -> (8.3194, -11.8759)
  arc A72 (8.3194, -11.8759) -> (8.7239, -11.5821) centre (0, 0) ccw
  line L73 (8.7239, -11.5821) -> (9.6396, -12.2971)
  arc A73 (9.6396, -12.2971) -> (10.0242, -11.9857) centre (0, 0) ccw
  line L74 (10.0242, -11.9857) -> (9.5152, -10.9413)
  arc A74 (9.5152, -10.9413) -> (9.8867, -10.6067) centre (0, 0) ccw
  line L75 (9.8867, -10.6067) -> (10.8722, -11.2221)
  arc A75 (10.8722, -11.2221) -> (11.2221, -10.8722) centre (0, 0) ccw
  line L76 (11.2221, -10.8722) -> (10.6067, -9.8867)
  arc A76 (10.6067, -9.8867) -> (10.9413, -9.5152) centre (0, 0) ccw
  line L77 (10.9413, -9.5152) -> (11.9857, -10.0242)
  arc A77 (11.9857, -10.0242) -> (12.2971, -9.6396) centre (0, 0) ccw
  line L78 (12.2971, -9.6396) -> (11.5821, -8.7239)
  arc A78 (11.5821, -8.7239) -> (11.8759, -8.3194) centre (0, 0) ccw
  line L79 (11.8759, -8.3194) -> (12.9678, -8.7165)
  arc A79 (12.9678, -8.7165) -> (13.2374, -8.3014) centre (0, 0) ccw
  line L80 (13.2374, -8.3014) -> (12.4305, -7.4654)
  arc A80 (12.4305, -7.4654) -> (12.6805, -7.0324) centre (0, 0) ccw
  line L81 (12.6805, -7.0324) -> (13.8079, -7.3132)
  arc A81 (13.8079, -7.3132) -> (14.0326, -6.8722) centre (0, 0) ccw
  line L82 (14.0326, -6.8722) -> (13.1428, -6.1252)
  arc A82 (13.1428, -6.1252) -> (13.3461, -5.6684) centre (0, 0) ccw
  line L83 (13.3461, -5.6684) -> (14.4967, -5.8298)
  arc A83 (14.4967, -5.8298) -> (14.674, -5.3678) centre (0, 0) ccw
  line L84 (14.674, -5.3678) -> (13.711, -4.7178)
  arc A84 (13.711, -4.7178) -> (13.8655, -4.2423) centre (0, 0) ccw
  line L85 (13.8655, -4.2423) -> (15.0267, -4.2826)
  arc A85 (15.0267, -4.2826) -> (15.1547, -3.8045) centre (0, 0) ccw
  line L86 (15.1547, -3.8045) -> (14.1291, -3.2588)
  arc A86 (14.1291, -3.2588) -> (14.233, -2.7697) centre (0, 0) ccw
  line L87 (14.233, -2.7697) -> (15.392, -2.6884)
  arc A87 (15.392, -2.6884) -> (15.4694, -2.1996) centre (0, 0) ccw
  line L88 (15.4694, -2.1996) -> (14.3923, -1.7641)
  arc A88 (14.3923, -1.7641) -> (14.4446, -1.2668) centre (0, 0) ccw
  line L89 (14.4446, -1.2668) -> (15.5887, -1.0648)
  arc A89 (15.5887, -1.0648) -> (15.6146, -0.5705) centre (0, 0) ccw
  line L90 (15.6146, -0.5705) -> (14.4978, -0.25)
  arc A90 (14.4978, -0.25) -> (14.4978, 0.25) centre (0, 0) ccw
  line L91 (14.4978, 0.25) -> (15.6146, 0.5705)
  arc A91 (15.6146, 0.5705) -> (15.5887, 1.0648) centre (0, 0) ccw
  line L92 (15.5887, 1.0648) -> (14.4446, 1.2668)
  arc A92 (14.4446, 1.2668) -> (14.3923, 1.7641) centre (0, 0) ccw
  line L93 (14.3923, 1.7641) -> (15.4694, 2.1996)
  arc A93 (15.4694, 2.1996) -> (15.392, 2.6884) centre (0, 0) ccw
  line L94 (15.392, 2.6884) -> (14.233, 2.7697)
  arc A94 (14.233, 2.7697) -> (14.1291, 3.2588) centre (0, 0) ccw
  line L95 (14.1291, 3.2588) -> (15.1547, 3.8045)
  arc A95 (15.1547, 3.8045) -> (15.0267, 4.2826) centre (0, 0) ccw
  line L96 (15.0267, 4.2826) -> (13.8655, 4.2423)
  arc A96 (13.8655, 4.2423) -> (13.711, 4.7178) centre (0, 0) ccw
  line L97 (13.711, 4.7178) -> (14.674, 5.3678)
  arc A97 (14.674, 5.3678) -> (14.4967, 5.8298) centre (0, 0) ccw
  line L98 (14.4967, 5.8298) -> (13.3461, 5.6684)
  arc A98 (13.3461, 5.6684) -> (13.1428, 6.1252) centre (0, 0) ccw
  line L99 (13.1428, 6.1252) -> (14.0326, 6.8722)
  arc A99 (14.0326, 6.8722) -> (13.8079, 7.3132) centre (0, 0) ccw
  line L100 (13.8079, 7.3132) -> (12.6805, 7.0324)
  arc A100 (12.6805, 7.0324) -> (12.4305, 7.4654) centre (0, 0) ccw
  line L101 (12.4305, 7.4654) -> (13.2374, 8.3014)
  arc A101 (13.2374, 8.3014) -> (12.9678, 8.7165) centre (0, 0) ccw
  line L102 (12.9678, 8.7165) -> (11.8759, 8.3194)
  arc A102 (11.8759, 8.3194) -> (11.5821, 8.7239) centre (0, 0) ccw
  line L103 (11.5821, 8.7239) -> (12.2971, 9.6396)
  arc A103 (12.2971, 9.6396) -> (11.9857, 10.0242) centre (0, 0) ccw
  line L104 (11.9857, 10.0242) -> (10.9413, 9.5152)
  arc A104 (10.9413, 9.5152) -> (10.6067, 9.8867) centre (0, 0) ccw
  line L105 (10.6067, 9.8867) -> (11.2221, 10.8722)
  arc A105 (11.2221, 10.8722) -> (10.8722, 11.2221) centre (0, 0) ccw
  line L106 (10.8722, 11.2221) -> (9.8867, 10.6067)
  arc A106 (9.8867, 10.6067) -> (9.5152, 10.9413) centre (0, 0) ccw
  line L107 (9.5152, 10.9413) -> (10.0242, 11.9857)
  arc A107 (10.0242, 11.9857) -> (9.6396, 12.2971) centre (0, 0) ccw
  line L108 (9.6396, 12.2971) -> (8.7239, 11.5821)
  arc A108 (8.7239, 11.5821) -> (8.3194, 11.8759) centre (0, 0) ccw
  line L109 (8.3194, 11.8759) -> (8.7165, 12.9678)
  arc A109 (8.7165, 12.9678) -> (8.3014, 13.2374) centre (0, 0) ccw
  line L110 (8.3014, 13.2374) -> (7.4654, 12.4305)
  arc A110 (7.4654, 12.4305) -> (7.0324, 12.6805) centre (0, 0) ccw
  line L111 (7.0324, 12.6805) -> (7.3132, 13.8079)
  arc A111 (7.3132, 13.8079) -> (6.8722, 14.0326) centre (0, 0) ccw
  line L112 (6.8722, 14.0326) -> (6.1252, 13.1428)
  arc A112 (6.1252, 13.1428) -> (5.6684, 13.3461) centre (0, 0) ccw
  line L113 (5.6684, 13.3461) -> (5.8298, 14.4967)
  arc A113 (5.8298, 14.4967) -> (5.3678, 14.674) centre (0, 0) ccw
  line L114 (5.3678, 14.674) -> (4.7178, 13.711)
  arc A114 (4.7178, 13.711) -> (4.2423, 13.8655) centre (0, 0) ccw
  line L115 (4.2423, 13.8655) -> (4.2826, 15.0267)
  arc A115 (4.2826, 15.0267) -> (3.8045, 15.1547) centre (0, 0) ccw
  line L116 (3.8045, 15.1547) -> (3.2588, 14.1291)
  arc A116 (3.2588, 14.1291) -> (2.7697, 14.233) centre (0, 0) ccw
  line L117 (2.7697, 14.233) -> (2.6884, 15.392)
  arc A117 (2.6884, 15.392) -> (2.1996, 15.4694) centre (0, 0) ccw
  line L118 (2.1996, 15.4694) -> (1.7641, 14.3923)
  arc A118 (1.7641, 14.3923) -> (1.2668, 14.4446) centre (0, 0) ccw
  line L119 (1.2668, 14.4446) -> (1.0648, 15.5887)
  arc A119 (1.0648, 15.5887) -> (0.5705, 15.6146) centre (0, 0) ccw
  point P0 (0, 0)
  point P1 (0, 0)
  point P2 (23.0887, 3.6569)
  point P3 (-3.6569, 23.0887)
  point P4 (-23.0887, -3.6569)
  point P5 (3.6569, -23.0887)
  dimension "d9" = 360
  constraints: 240 end point, 240 point on circle, 120 centre point, 5 other
hole "Bohrung1" at (2, 3.6569, -23.0887) at (2, 23.0887, 3.6569) at (2, -3.6569, 23.0887) at (2, -23.0887, -3.6569) direction (-1, 0, 0) diameter 2.2 depth 4 tip angle 118 counterbore diameter 4 counterbore depth 2.2
sketch "Skizze5" plane through (2, 0, 0) normal (1, 0, 0) x (0, 0, -1)
  circle A0 centre (-3.6569, 23.0887) radius 1.1 projected
  line L0 (-1.5828, 23.4173) -> (-1.8229, 24.9335)
  line L1 (-5.9712, 24.2764) -> (-5.731, 22.7602)
  arc A1 (-5.731, 22.7602) -> (-1.5828, 23.4173) centre (-3.6569, 23.0887) ccw
  circle A2 centre (0, 0) radius 25
  line L2 (-23.4173, -1.5828) -> (-24.9335, -1.8229)
  line L3 (-24.2764, -5.9712) -> (-22.7602, -5.731)
  arc A3 (-22.7602, -5.731) -> (-23.4173, -1.5828) centre (-23.0887, -3.6569) ccw
  line L4 (1.5828, -23.4173) -> (1.8229, -24.9335)
  line L5 (5.9712, -24.2764) -> (5.731, -22.7602)
  arc A4 (5.731, -22.7602) -> (1.5828, -23.4173) centre (3.6569, -23.0887) ccw
  line L6 (23.4173, 1.5828) -> (24.9335, 1.8229)
  line L7 (24.2764, 5.9712) -> (22.7602, 5.731)
  arc A5 (22.7602, 5.731) -> (23.4173, 1.5828) centre (23.0887, 3.6569) ccw
  point P0 (-3.9149, 24.718)
  point P1 (-24.718, -3.9149)
  point P2 (3.9149, -24.718)
  point P3 (24.718, 3.9149)
  dimension "d17" = 4.2
  dimension "d20" = 360
  constraints: 16 end point, 10 point on circle, 5 centre point, 2 tangent, 1 coincident, 1 parallel, 37 other
  measures "d17" distance between parallel lines of L1 L0
extrude "Extrusion2" cut sketch "Skizze5" against normal blind 2.2 contours A1 L1 A2 L0 | A2 L6 A5 L7 | L2 A3 L3 A2 | A2 L4 A4 L5
fillet "Rundung1" radius 1.5 8 edges at (0.9, -24.2764, -5.9712) (0.9, -24.9335, -1.8229) (0.9, 1.8229, -24.9335) (0.9, 5.9712, -24.2764) (0.9, 24.9335, 1.8229) (0.9, 24.2764, 5.9712) (0.9, -1.8229, 24.9335) (0.9, -5.9712, 24.2764)
body "Solid1"
